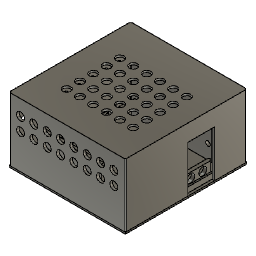
power hotbed caddy v6 (Autodesk Fusion 360 design; units mm, degrees)
Autodesk Fusion 360 part; units mm, degrees
sketch "OUTLINE" plane through (0, 0, 0) normal (0, 0, 1) x (1, 0, 0)
  line L0 (42, -44) -> (-42, -44)
  line L1 (-42, -44) -> (-42, 44)
  line L2 (-42, 44) -> (42, 44)
  line L3 (42, 44) -> (42, -44)
  line L4 (42, -44) -> (-42, 44) construction
  line L5 (-42, -44) -> (42, 44) construction
  line L6 (-42, -44) -> (-40.4, -44) construction
  line L7 (-40.4, -44) -> (-40.4, 44) construction
  line L8 (-40.4, 44) -> (-42, 44) construction
  line L9 (-42, 44) -> (-42, -44) construction
  line L10 (-42, -44) -> (42, -44) construction
  line L11 (42, -44) -> (42, -42.4) construction
  line L12 (42, -42.4) -> (-42, -42.4) construction
  line L13 (-42, -42.4) -> (-42, -44) construction
  line L14 (42, -44) -> (40.4, -44) construction
  line L15 (40.4, -44) -> (40.4, 44) construction
  line L16 (40.4, 44) -> (42, 44) construction
  line L17 (42, 44) -> (42, -44) construction
  line L18 (42, 44) -> (-42, 44) construction
  line L19 (-42, 44) -> (-42, 42.4) construction
  line L20 (-42, 42.4) -> (42, 42.4) construction
  line L21 (42, 42.4) -> (42, 44) construction
  line L22 (40.4, 42.3238) -> (-40.4, 42.3238)
  line L23 (-40.4, 42.3238) -> (-40.4, -42.3238)
  line L24 (-40.4, -42.3238) -> (40.4, -42.3238)
  line L25 (40.4, -42.3238) -> (40.4, 42.3238)
  line L26 (40.4, 42.3238) -> (-40.4, -42.3238) construction
  line L27 (-40.4, 42.3238) -> (40.4, -42.3238) construction
  line L28 (-40.4, -42.3238) -> (40.4, -42.3238) construction
  line L29 (40.4, -42.3238) -> (40.4, -34.3238) construction
  line L30 (40.4, -34.3238) -> (-40.4, -34.3238) construction
  line L31 (-40.4, -34.3238) -> (-40.4, -42.3238) construction
  line L32 (-40.4, 42.3238) -> (40.4, 42.3238) construction
  line L33 (40.4, 42.3238) -> (40.4, 34.3238) construction
  line L34 (40.4, 34.3238) -> (-40.4, 34.3238) construction
  line L35 (-40.4, 34.3238) -> (-40.4, 42.3238) construction
  line L36 (-29.5478, 34.3238) -> (30.4522, 34.3238)
  line L37 (30.4522, 34.3238) -> (30.4522, 32.3238)
  line L38 (30.4522, 32.3238) -> (-29.5478, 32.3238)
  line L39 (-29.5478, 32.3238) -> (-29.5478, 34.3238)
  line L40 (-29.5478, -34.3238) -> (14.4522, -34.3238)
  line L41 (14.4522, -34.3238) -> (14.4522, -32.3238)
  line L42 (14.4522, -32.3238) -> (-29.5478, -32.3238)
  line L43 (-29.5478, -32.3238) -> (-29.5478, -34.3238)
  line L44 (-36.5645, -28.9894) -> (-33.9645, -28.9894)
  line L45 (-33.9645, -28.9894) -> (-33.9645, 26.0106)
  line L46 (-33.9645, 26.0106) -> (-36.5645, 26.0106)
  line L47 (-36.5645, 26.0106) -> (-36.5645, -28.9894)
  line L48 (34.4355, 26.0106) -> (34.4355, -28.9894)
  line L49 (34.4355, -28.9894) -> (37.0355, -28.9894)
  line L50 (37.0355, -28.9894) -> (37.0355, 26.0106)
  line L51 (37.0355, 26.0106) -> (34.4355, 26.0106)
  line L52 (43.6, -45.6) -> (-43.6, -45.6)
  line L53 (-43.6, -45.6) -> (-43.6, 45.6)
  line L54 (-43.6, 45.6) -> (43.6, 45.6)
  line L55 (43.6, 45.6) -> (43.6, -45.6)
  line L56 (43.6, -45.6) -> (-43.6, 45.6) construction
  line L57 (-43.6, -45.6) -> (43.6, 45.6) construction
  dimension "d1" = 84
  dimension "d2" = 88
  dimension "d3" = 1.6
  dimension "d4" = 1.6
  dimension "d5" = 1.6
  dimension "d6" = 1.6
  dimension "d7" = 8
  dimension "d8" = 80.8
  dimension "d9" = 8
  dimension "d10" = 60
  dimension "d11" = 2
  dimension "d12" = 44
  dimension "d13" = 2
  dimension "d14" = 80.8
  dimension "d15" = 2.6
  dimension "d16" = 55
  dimension "d17" = 2.6
  dimension "d18" = 55
  dimension "d47" = 1.6
  dimension "d48" = 1.6
  constraint horizontal L0
  constraint perpendicular L0 L1
  constraint parallel L0 L2
  constraint parallel L1 L3
  constraint coincident L4 origin
  constraint coincident L5 origin
  constraint horizontal L6
  constraint vertical L7
  constraint horizontal L8
  constraint vertical L9
  constraint horizontal L10
  constraint vertical L11
  constraint horizontal L12
  constraint vertical L13
  constraint horizontal L14
  constraint vertical L15
  constraint horizontal L16
  constraint vertical L17
  constraint horizontal L18
  constraint vertical L19
  constraint horizontal L20
  constraint vertical L21
  constraint horizontal L22
  constraint perpendicular L22 L23
  constraint parallel L22 L24
  constraint parallel L23 L25
  constraint coincident L5 L22.start
  constraint coincident L15 L22.start
  constraint coincident L26 origin
  constraint coincident L27 origin
  constraint horizontal L28
  constraint vertical L29
  constraint horizontal L30
  constraint vertical L31
  constraint horizontal L32
  constraint vertical L33
  constraint horizontal L34
  constraint vertical L35
  constraint horizontal L36
  constraint vertical L37
  constraint horizontal L38
  constraint vertical L39
  constraint coincident L34 L36.start
  constraint horizontal L40
  constraint vertical L41
  constraint horizontal L42
  constraint vertical L43
  constraint coincident L30 L40.start
  constraint horizontal L44
  constraint vertical L45
  constraint horizontal L46
  constraint vertical L47
  constraint horizontal L49
  constraint vertical L50
  constraint horizontal L51
  constraint vertical L48
  constraint horizontal L52
  constraint perpendicular L52 L53
  constraint parallel L52 L54
  constraint parallel L53 L55
  constraint coincident L56 origin
  constraint coincident L57 origin
  measures "d1" distance of L1.end L2.end
  measures "d2" distance of L0.end L1.end
  measures "d3" distance of L0.end L6.end
  measures "d4" distance of L0.end L12.end
  measures "d5" distance of L0.start L14.end
  measures "d6" distance of L2.end L20.end
  measures "d7" distance of L23.end L30.end
  measures "d8" distance of L22.end L22.start
  measures "d9" distance of L22.end L34.end
  measures "d10" distance of L36.start L36.end
  measures "d11" distance of L36.start L38.end
  measures "d12" distance of L40.start L40.end
  measures "d13" distance of L40.start L42.end
  measures "d14" distance of L29.end L30.end
  measures "d15" distance of L44.start L44.end
  measures "d16" distance of L44.start L46.end
  measures "d17" distance of L49.end L48.end
  measures "d18" distance of L48.end L48.start
  measures "d47" distance of L3 L55
  measures "d48" distance of L10 L52
extrude "Extrude1" add sketch "OUTLINE" against normal blind 1 contours L0 L1 L2 L3 | L22 L23 L24 L25 | L36 L37 L38 L39 | L40 L41 L42 L43 | L44 L45 L46 L47 | L48 L49 L50 L51 makes body 1
extrude "Extrude2" add sketch "OUTLINE" along normal blind 44 contours L36 L37 L38 L39 bodies 1
extrude "Extrude3" add sketch "OUTLINE" along normal blind 24 contours L40 L41 L42 L43 bodies 1
extrude "Extrude4" add sketch "OUTLINE" along normal blind 8 contours L48 L49 L50 L51 bodies 1
extrude "Extrude5" add sketch "OUTLINE" along normal blind 8 contours L44 L45 L46 L47 bodies 1
hole "Hole1" at (-36.5645, 19.0841, 3.9854) direction (1, 0, 0) diameter 6 depth 100 tip angle 118 bodies 1
hole "Hole2" at (-36.5645, 10.019, 4.0988) direction (1, 0, 0) diameter 6 depth 100 tip angle 118 bodies 1
hole "Hole3" at (-36.5645, 1.1791, 4.164) direction (1, 0, 0) diameter 6 depth 100 tip angle 118 bodies 1
hole "Hole4" at (-36.5645, -7.2432, 4.1822) direction (1, 0, 0) diameter 6 depth 100 tip angle 118 bodies 1
hole "Hole5" at (-36.5645, -14.9986, 4.2656) direction (1, 0, 0) diameter 6 depth 100 tip angle 118 bodies 1
hole "Hole6" at (-36.5645, -22.5039, 4.0988) direction (1, 0, 0) diameter 6 depth 100 tip angle 118 bodies 1
extrude "Extrude6" add sketch "OUTLINE" along normal blind 2 contours L0 L1 L2 L3 bodies 1
extrude "Extrude7" add sketch "OUTLINE" along normal blind 46 separate body contours L52 L53 L54 L55 makes body 2
extrude "Extrude8" add sketch "OUTLINE" against normal blind 1 contours L52 L53 L54 L55 bodies 1
extrude "Extrude9" cut 1 faces at (-42, -14.6667, 0.6667) along direction (1, 0, 0) blind 0.4 on bodies 1 bodies 1
extrude "Extrude10" cut 1 faces at (14.1333, -44, 0.6667) along direction (0, 1, 0) blind 0.4 on bodies 1 bodies 1
extrude "Extrude12" cut 1 faces at (42, 14.8, 0.6667) along direction (-1, 0, 0) blind 0.4 on bodies 1 bodies 1
extrude "Extrude13" cut 1 faces at (-13.8667, 44, 0.6667) along direction (0, -1, 0) blind 0.4 on bodies 1 bodies 1
chamfer "Chamfer1" distance 1 angle 45 1 edges at (41.6, -43.6, 1) on bodies 1
chamfer "Chamfer2" distance 1 angle 45 1 edges at (-41.6, -43.6, 1) on bodies 1
chamfer "Chamfer3" distance 1 angle 45 1 edges at (-41.6, 43.6, 1) on bodies 1
chamfer "Chamfer4" distance 1 angle 45 1 edges at (41.6, 43.6, 1) on bodies 1
chamfer "Chamfer5" distance 1 angle 45 2 edges at (37.0355, 26.0106, 4) (34.4355, 26.0106, 4) on bodies 1
chamfer "Chamfer6" distance 1 angle 45 2 edges at (37.0355, -28.9894, 4) (34.4355, -28.9894, 4) on bodies 1
chamfer "Chamfer7" distance 1 angle 45 4 edges at (-33.9645, -28.9894, 4) (-36.5645, -28.9894, 4) (-36.5645, 26.0106, 4) (-33.9645, 26.0106, 4) on bodies 1
sketch "TOP" plane through (0, 0, 46) normal (0, 0, 1) x (-1, 0, 0)
  line L0 (42, -44) -> (-42, -44)
  line L1 (-42, -44) -> (-42, 44)
  line L2 (-42, 44) -> (42, 44)
  line L3 (42, 44) -> (42, -44)
  line L4 (-43.6, -45.6) -> (43.6, -45.6)
  line L5 (43.6, -45.6) -> (43.6, 45.6)
  line L6 (43.6, 45.6) -> (-43.6, 45.6)
  line L7 (-43.6, 45.6) -> (-43.6, -45.6)
  line L8 (43.6, -45.6) -> (-43.6, -45.6)
  line L9 (-43.6, -45.6) -> (-43.6, 45.6)
  line L10 (-43.6, 45.6) -> (43.6, 45.6)
  line L11 (43.6, 45.6) -> (43.6, -45.6)
  constraint horizontal L8
  constraint vertical L9
  constraint horizontal L10
  constraint vertical L11
  constraint coincident L6.end L7.start
  constraint coincident L4.end L5.start
extrude "Extrude14" add sketch "TOP" along normal blind 1.2 contours L0 L1 L2 L3 | L4 L5 L6 L7 L8 L9 L10 L11 bodies 2
sketch "CABLE HOLES" plane through (-43.6, 0, 0) normal (-1, 0, 0) x (0, -1, 0)
  line L0 (-45.6, 0) -> (45.6, 0)
  line L1 (45.6, 0) -> (45.6, 47.2)
  line L2 (45.6, 47.2) -> (-45.6, 47.2)
  line L3 (-45.6, 47.2) -> (-45.6, 0)
  line L4 (-21.3761, 35, -87.2) -> (-1.3761, 35, -87.2)
  line L5 (-1.3761, 35, -87.2) -> (-1.3761, 0, -87.2)
  line L6 (-1.3761, 0, -87.2) -> (-21.3761, 0, -87.2)
  line L7 (-21.3761, 0, -87.2) -> (-21.3761, 35, -87.2)
  dimension "d74" = 20
  dimension "d75" = 35
extrude "Extrude15" [suppressed]
sketch "BUCK CONVERTER MOUNTING" plane through (0, -34.3238, 0) normal (0, -1, 0) x (1, 0, 0)
  line L0 (-29.5478, 0) -> (14.4522, 0)
  line L1 (14.4522, 0) -> (14.4522, 24)
  line L2 (14.4522, 24) -> (-29.5478, 24)
  line L3 (-29.5478, 24) -> (-29.5478, 0)
  line L4 (-29.5478, 24) -> (-28.5478, 24) construction
  line L5 (-28.5478, 24) -> (-28.5478, 4) construction
  line L6 (-28.5478, 4) -> (-29.5478, 4) construction
  line L7 (-29.5478, 4) -> (-29.5478, 24) construction
  line L8 (14.4522, 24) -> (13.4522, 24) construction
  line L9 (13.4522, 24) -> (13.4522, 4) construction
  line L10 (13.4522, 4) -> (14.4522, 4) construction
  line L11 (14.4522, 4) -> (14.4522, 24) construction
  line L12 (-29.5478, 24) -> (-24.5478, 24) construction
  line L13 (-24.5478, 24) -> (-24.5478, 23) construction
  line L14 (-24.5478, 23) -> (-29.5478, 23) construction
  line L15 (-29.5478, 23) -> (-29.5478, 24) construction
  line L16 (-29.5478, 4) -> (-24.5478, 4) construction
  line L17 (-24.5478, 4) -> (-24.5478, 5) construction
  line L18 (-24.5478, 5) -> (-29.5478, 5) construction
  line L19 (-29.5478, 5) -> (-29.5478, 4) construction
  line L20 (14.4522, 24) -> (9.4522, 24) construction
  line L21 (9.4522, 24) -> (9.4522, 23) construction
  line L22 (9.4522, 23) -> (14.4522, 23) construction
  line L23 (14.4522, 23) -> (14.4522, 24) construction
  line L24 (14.4522, 4) -> (9.4522, 4) construction
  line L25 (9.4522, 4) -> (9.4522, 5) construction
  line L26 (9.4522, 5) -> (14.4522, 5) construction
  line L27 (14.4522, 5) -> (14.4522, 4) construction
  circle A0 centre (-22.7778, 21.23) radius 1.77
  circle A1 centre (7.6822, 21.23) radius 1.77
  circle A2 centre (7.6822, 6.77) radius 1.77
  circle A3 centre (-22.7778, 6.77) radius 1.77
  dimension "d78" = 1
  dimension "d79" = 20
  dimension "d80" = 1
  dimension "d81" = 20
  dimension "d82" = 5
  dimension "d83" = 1
  dimension "d84" = 5
  dimension "d85" = 1
  dimension "d86" = 5
  dimension "d87" = 1
  dimension "d88" = 5
  dimension "d89" = 1
  dimension "d90" = 1.77
  dimension "d91" = 1.77
  dimension "d92" = 1.77
  dimension "d93" = 1.77
  constraint horizontal L4
  constraint vertical L5
  constraint horizontal L6
  constraint vertical L7
  constraint coincident L2.end L3.start
  constraint horizontal L8
  constraint vertical L9
  constraint horizontal L10
  constraint vertical L11
  constraint coincident L1.end L2.start
  constraint horizontal L12
  constraint vertical L13
  constraint horizontal L14
  constraint vertical L15
  constraint horizontal L16
  constraint vertical L17
  constraint horizontal L18
  constraint vertical L19
  constraint horizontal L20
  constraint vertical L21
  constraint horizontal L22
  constraint vertical L23
  constraint horizontal L24
  constraint vertical L25
  constraint horizontal L26
  constraint vertical L27
  constraint tangent L14 A0
  constraint tangent L13 A0
  constraint tangent L21 A1
  constraint tangent L22 A1
  constraint tangent L25 A2
  constraint tangent L26 A2
  constraint tangent L17 A3
  constraint tangent L18 A3
  measures "d78" distance of L2.end L4.end
  measures "d79" distance of L2.end L6.end
  measures "d80" distance of L1.end L8.end
  measures "d81" distance of L1.end L10.end
  measures "d82" distance of L2.end L12.end
  measures "d83" distance of L2.end L14.end
  measures "d84" distance of L6.end L16.end
  measures "d85" distance of L6.end L18.end
  measures "d86" distance of L1.end L20.end
  measures "d87" distance of L1.end L22.end
  measures "d88" distance of L10.end L24.end
  measures "d89" distance of L10.end L26.end
  measures "d90" radius of A0
  measures "d91" radius of A1
  measures "d92" radius of A2
  measures "d93" radius of A3
sketch "HOTBED POWER MODULE MOUNTING" plane through (0, 32.3238, 0) normal (0, -1, 0) x (1, 0, 0)
  line L0 (-29.5478, 0) -> (30.4522, 0)
  line L1 (30.4522, 0) -> (30.4522, 44)
  line L2 (30.4522, 44) -> (-29.5478, 44)
  line L3 (-29.5478, 44) -> (-29.5478, 0)
  line L4 (-29.5478, 44) -> (-28.5478, 44) construction
  line L5 (-28.5478, 44) -> (-28.5478, 4) construction
  line L6 (-28.5478, 4) -> (-29.5478, 4) construction
  line L7 (-29.5478, 4) -> (-29.5478, 44) construction
  line L8 (30.4522, 44) -> (29.4522, 44) construction
  line L9 (29.4522, 44) -> (29.4522, 4) construction
  line L10 (29.4522, 4) -> (30.4522, 4) construction
  line L11 (30.4522, 4) -> (30.4522, 44) construction
  line L12 (-29.5478, 44) -> (-28.5478, 44) construction
  line L13 (-28.5478, 44) -> (-28.5478, 39) construction
  line L14 (-28.5478, 39) -> (-29.5478, 39) construction
  line L15 (-29.5478, 39) -> (-29.5478, 44) construction
  line L16 (30.4522, 44) -> (29.4522, 44) construction
  line L17 (29.4522, 44) -> (29.4522, 39) construction
  line L18 (29.4522, 39) -> (30.4522, 39) construction
  line L19 (30.4522, 39) -> (30.4522, 44) construction
  line L20 (30.4522, 4) -> (29.4522, 4) construction
  line L21 (29.4522, 4) -> (29.4522, 9) construction
  line L22 (29.4522, 9) -> (30.4522, 9) construction
  line L23 (30.4522, 9) -> (30.4522, 4) construction
  line L24 (-29.5478, 4) -> (-28.5478, 4) construction
  line L25 (-28.5478, 4) -> (-28.5478, 9) construction
  line L26 (-28.5478, 9) -> (-29.5478, 9) construction
  line L27 (-29.5478, 9) -> (-29.5478, 4) construction
  line L28 (-28.5478, 24) -> (-28.5478, 4)
  circle A0 centre (-26.7778, 10.77) radius 1.77
  circle A1 centre (27.6822, 10.77) radius 1.77
  circle A2 centre (-26.7778, 37.23) radius 1.77
  circle A3 centre (27.6822, 37.23) radius 1.77
  dimension "d94" = 1
  dimension "d95" = 40
  dimension "d96" = 1
  dimension "d97" = 40
  dimension "d98" = 1
  dimension "d99" = 5
  dimension "d100" = 1
  dimension "d101" = 5
  dimension "d102" = 1
  dimension "d103" = 5
  dimension "d104" = 1
  dimension "d105" = 5
  dimension "d106" = 1.77
  dimension "d107" = 1.77
  dimension "d108" = 1.77
  dimension "d109" = 1.77
  constraint horizontal L4
  constraint vertical L5
  constraint horizontal L6
  constraint vertical L7
  constraint coincident L2.end L3.start
  constraint horizontal L8
  constraint vertical L9
  constraint horizontal L10
  constraint vertical L11
  constraint coincident L1.end L2.start
  constraint horizontal L12
  constraint vertical L13
  constraint horizontal L14
  constraint vertical L15
  constraint horizontal L16
  constraint vertical L17
  constraint horizontal L18
  constraint vertical L19
  constraint horizontal L20
  constraint vertical L21
  constraint horizontal L22
  constraint vertical L23
  constraint horizontal L24
  constraint vertical L25
  constraint horizontal L26
  constraint vertical L27
  constraint tangent L28 A0
  constraint tangent L26 A0
  constraint tangent L21 A1
  constraint tangent L22 A1
  constraint tangent L14 A2
  constraint tangent L5 A2
  constraint tangent L9 A3
  constraint tangent L18 A3
  measures "d94" distance of L2.end L4.end
  measures "d95" distance of L2.end L6.end
  measures "d96" distance of L1.end L8.end
  measures "d97" distance of L1.end L10.end
  measures "d98" distance of L2.end L4.end
  measures "d99" distance of L2.end L14.end
  measures "d100" distance of L1.end L8.end
  measures "d101" distance of L1.end L18.end
  measures "d102" distance of L10.end L9.end
  measures "d103" distance of L10.end L22.end
  measures "d104" distance of L6.end L5.end
  measures "d105" distance of L6.end L26.end
  measures "d106" radius of A0
  measures "d107" radius of A1
  measures "d108" radius of A2
  measures "d109" radius of A3
extrude "Extrude16" cut sketch "HOTBED POWER MODULE MOUNTING" against normal blind 6 contours A0 | A1 | A2 | A3 bodies 1
extrude "Extrude17" cut sketch "BUCK CONVERTER MOUNTING" against normal blind 9 contours A0 | A1 | A2 | A3 bodies 1
sketch "SIDE HOLES (1)" plane through (-43.6, 0, 0) normal (-1, 0, 0) x (0, -1, 0)
  line L0 (-45.6, 0) -> (45.6, 0)
  line L1 (45.6, 0) -> (45.6, 47.2)
  line L2 (45.6, 47.2) -> (-45.6, 47.2)
  line L3 (-45.6, 47.2) -> (-45.6, 0)
  circle A0 centre (-34, 36) radius 3
  circle A1 centre (-34, 26) radius 3
  circle A2 centre (-24, 26) radius 3
  circle A3 centre (-24, 36) radius 3
  circle A4 centre (-14, 26) radius 3
  circle A5 centre (-14, 36) radius 3
  circle A6 centre (-4, 36) radius 3
  circle A7 centre (-4, 26) radius 3
  circle A8 centre (6, 36) radius 3
  circle A9 centre (6, 26) radius 3
  circle A10 centre (16, 26) radius 3
  circle A11 centre (16, 36) radius 3
  circle A12 centre (26, 36) radius 3
  circle A13 centre (26, 26) radius 3
  circle A14 centre (36, 26) radius 3
  circle A15 centre (36, 36) radius 3
  dimension "d114" = 6
  dimension "d115" = 6
  dimension "d116" = 6
  dimension "d117" = 6
  dimension "d118" = 6
  dimension "d119" = 6
  dimension "d120" = 6
  dimension "d121" = 6
  dimension "d122" = 6
  dimension "d123" = 6
  dimension "d124" = 6
  dimension "d125" = 6
  dimension "d126" = 6
  dimension "d127" = 6
  dimension "d128" = 6
  dimension "d129" = 6
  measures "d114" diameter of A0
  measures "d115" diameter of A1
  measures "d116" diameter of A3
  measures "d117" diameter of A2
  measures "d118" diameter of A5
  measures "d119" diameter of A4
  measures "d120" diameter of A6
  measures "d121" diameter of A7
  measures "d122" diameter of A8
  measures "d123" diameter of A9
  measures "d124" diameter of A11
  measures "d125" diameter of A10
  measures "d126" diameter of A12
  measures "d127" diameter of A13
  measures "d128" diameter of A15
  measures "d129" diameter of A14
extrude "Extrude18" cut sketch "SIDE HOLES (1)" against normal blind 7 contours A0 | A1 | A2 | A3 | A4 | A5 | A6 | A7 | A8 | A9 | A10 | A11 | A12 | A13 | A14 | A15 bodies 2
sketch "OTHER SIDE HOLES" plane through (0, -45.6, 0) normal (0, -1, 0) x (1, 0, 0)
  line L0 (-43.6, 0) -> (43.6, 0)
  line L1 (43.6, 0) -> (43.6, 47.2)
  line L2 (43.6, 47.2) -> (-43.6, 47.2)
  line L3 (-43.6, 47.2) -> (-43.6, 0)
  circle A0 centre (-35, 36) radius 3
  circle A1 centre (-25, 36) radius 3
  circle A2 centre (-15, 36) radius 3
  circle A3 centre (-5, 36) radius 3
  circle A4 centre (5, 36) radius 3
  circle A5 centre (15, 36) radius 3
  circle A6 centre (25, 36) radius 3
  circle A7 centre (35, 36) radius 3
  circle A8 centre (-35, 26) radius 3
  circle A9 centre (-25, 26) radius 3
  circle A10 centre (-15, 26) radius 3
  circle A11 centre (-5, 26) radius 3
  circle A12 centre (5, 26) radius 3
  circle A13 centre (15, 26) radius 3
  circle A14 centre (25, 26) radius 3
  circle A15 centre (35, 26) radius 3
  dimension "d132" = 6
  dimension "d133" = 6
  dimension "d134" = 6
  dimension "d135" = 6
  dimension "d136" = 6
  dimension "d137" = 6
  dimension "d138" = 6
  dimension "d139" = 6
  dimension "d140" = 6
  dimension "d141" = 6
  dimension "d142" = 6
  dimension "d143" = 6
  dimension "d144" = 6
  dimension "d145" = 6
  dimension "d146" = 6
  dimension "d147" = 6
  measures "d132" diameter of A0
  measures "d133" diameter of A1
  measures "d134" diameter of A2
  measures "d135" diameter of A3
  measures "d136" diameter of A4
  measures "d137" diameter of A5
  measures "d138" diameter of A6
  measures "d139" diameter of A7
  measures "d140" diameter of A8
  measures "d141" diameter of A9
  measures "d142" diameter of A10
  measures "d143" diameter of A11
  measures "d144" diameter of A12
  measures "d145" diameter of A13
  measures "d146" diameter of A14
  measures "d147" diameter of A15
extrude "Extrude19" cut sketch "OTHER SIDE HOLES" against normal blind 118 contours A0 | A1 | A2 | A3 | A4 | A5 | A6 | A7 | A8 | A9 | A10 | A11 | A12 | A13 | A14 | A15 bodies 2
chamfer "Chamfer8" distance 1 angle 45 2 edges at (43.6, -45.6, 23.6) (43.6, 45.6, 23.6) on bodies 2
sketch "top holes" plane through (0, 0, 47.2) normal (0, 0, 1) x (-1, 0, 0)
  line L0 (-42.6, -45.6) -> (43.6, -45.6)
  line L1 (43.6, -45.6) -> (43.6, 45.6)
  line L2 (43.6, 45.6) -> (-42.6, 45.6)
  line L3 (-43.6, 44.6) -> (-43.6, -44.6)
  circle A0 centre (-26, -18) radius 3
  circle A1 centre (-26, -8) radius 3
  circle A2 centre (-26, 2) radius 3
  circle A3 centre (-26, 12) radius 3
  circle A4 centre (-26, 22) radius 3
  circle A5 centre (-16, -8) radius 3
  circle A6 centre (-16, -18) radius 3
  circle A7 centre (-16, 2) radius 3
  circle A8 centre (-16, 12) radius 3
  circle A9 centre (-16, 22) radius 3
  circle A10 centre (4, -18) radius 3
  circle A11 centre (4, -8) radius 3
  circle A12 centre (4, 2) radius 3
  circle A13 centre (4, 12) radius 3
  circle A14 centre (4, 22) radius 3
  circle A15 centre (-6, 22) radius 3
  circle A16 centre (-6, 12) radius 3
  circle A17 centre (-6, 2) radius 3
  circle A18 centre (-6, -8) radius 3
  circle A19 centre (-6, -18) radius 3
  circle A20 centre (14, -18) radius 3
  circle A21 centre (14, -8) radius 3
  circle A22 centre (14, 2) radius 3
  circle A23 centre (14, 12) radius 3
  circle A24 centre (14, 22) radius 3
  circle A25 centre (24, 22) radius 3
  circle A26 centre (24, 12) radius 3
  circle A27 centre (24, 2) radius 3
  circle A28 centre (24, -8) radius 3
  circle A29 centre (24, -18) radius 3
  line L4 (-43.6, -44.6) -> (-42.6, -45.6)
  line L5 (-42.6, 45.6) -> (-43.6, 44.6)
  dimension "d151" = 6
  dimension "d152" = 6
  dimension "d153" = 6
  dimension "d154" = 6
  dimension "d155" = 6
  dimension "d156" = 6
  dimension "d157" = 6
  dimension "d158" = 6
  dimension "d159" = 6
  dimension "d160" = 6
  dimension "d161" = 10
  dimension "d162" = 10
  dimension "d163" = 10
  dimension "d164" = 10
  dimension "d165" = 10
  dimension "d166" = 6
  dimension "d167" = 6
  dimension "d168" = 6
  dimension "d169" = 6
  dimension "d170" = 6
  dimension "d171" = 6
  dimension "d172" = 6
  dimension "d173" = 6
  dimension "d174" = 6
  dimension "d175" = 6
  dimension "d176" = 10
  dimension "d177" = 10
  dimension "d178" = 10
  dimension "d179" = 10
  dimension "d180" = 10
  dimension "d181" = 6
  dimension "d182" = 6
  dimension "d183" = 6
  dimension "d184" = 6
  dimension "d185" = 6
  dimension "d186" = 6
  dimension "d187" = 6
  dimension "d188" = 6
  dimension "d189" = 6
  dimension "d190" = 6
  dimension "d191" = 10
  dimension "d192" = 10
  dimension "d193" = 10
  dimension "d194" = 10
  dimension "d195" = 10
  measures "d151" diameter of A0
  measures "d152" diameter of A1
  measures "d153" diameter of A2
  measures "d154" diameter of A3
  measures "d155" diameter of A4
  measures "d156" diameter of A6
  measures "d157" diameter of A5
  measures "d158" diameter of A7
  measures "d159" diameter of A8
  measures "d160" diameter of A9
  measures "d161" distance of A0.centre A6.centre
  measures "d162" distance of A1.centre A5.centre
  measures "d163" distance of A2.centre A7.centre
  measures "d164" distance of A3.centre A8.centre
  measures "d165" distance of A4.centre A9.centre
  measures "d166" diameter of A19
  measures "d167" diameter of A18
  measures "d168" diameter of A17
  measures "d169" diameter of A16
  measures "d170" diameter of A15
  measures "d171" diameter of A10
  measures "d172" diameter of A11
  measures "d173" diameter of A12
  measures "d174" diameter of A13
  measures "d175" diameter of A14
  measures "d176" distance of A19.centre A10.centre
  measures "d177" distance of A18.centre A11.centre
  measures "d178" distance of A12.centre A17.centre
  measures "d179" distance of A16.centre A13.centre
  measures "d180" distance of A15.centre A14.centre
  measures "d181" diameter of A20
  measures "d182" diameter of A21
  measures "d183" diameter of A22
  measures "d184" diameter of A23
  measures "d185" diameter of A24
  measures "d186" diameter of A29
  measures "d187" diameter of A28
  measures "d188" diameter of A27
  measures "d189" diameter of A26
  measures "d190" diameter of A25
  measures "d191" distance of A20.centre A29.centre
  measures "d192" distance of A21.centre A28.centre
  measures "d193" distance of A27.centre A22.centre
  measures "d194" distance of A23.centre A26.centre
  measures "d195" distance of A24.centre A25.centre
extrude "Extrude20" cut sketch "top holes" against normal blind 2 contours A0 | A1 | A2 | A3 | A4 | A5 | A6 | A7 | A8 | A9 | A10 | A11 | A12 | A13 | A14 | A15 | A16 | A17 | A18 | A19 | A20 | A21 | A22 | A23 | A24 | A25 | A26 | A27 | A28 | A29 bodies 2
extrude "Extrude21" cut sketch "CABLE HOLES" along normal blind 2 contours L4 L5 L6 L7 in plane through (43.6, 0, 0) normal (-1, 0, 0) bodies 2
sketch "Sketch10" plane through (-43.6, 0, 0) normal (-1, 0, 0) x (0, -1, 0)
  circle A0 centre (-14, 36) radius 3
  circle A1 centre (-14, 26) radius 3
  circle A2 centre (26, 26) radius 3
  circle A3 centre (16, 36) radius 3
  circle A4 centre (26, 36) radius 3
  circle A5 centre (16, 26) radius 3
  circle A6 centre (-24, 26) radius 3
  circle A7 centre (-4, 36) radius 3
  circle A8 centre (-24, 36) radius 3
  circle A9 centre (-4, 26) radius 3
  circle A10 centre (36, 26) radius 3
  circle A11 centre (-34, 36) radius 3
  circle A12 centre (36, 36) radius 3
  circle A13 centre (6, 26) radius 3
  circle A14 centre (-34, 26) radius 3
  circle A15 centre (6, 36) radius 3
  line L0 (-45.6, 0) -> (45.6, 0)
  line L1 (45.6, 0) -> (45.6, 47.2)
  line L2 (45.6, 47.2) -> (-45.6, 47.2)
  line L3 (-45.6, 47.2) -> (-45.6, 0)
  line L4 (-8, 0) -> (2, 0)
  line L5 (2, 0) -> (2, 15)
  line L6 (2, 15) -> (-8, 15)
  line L7 (-8, 15) -> (-8, 0)
  dimension "d200" = 10
  dimension "d201" = 15
  constraint horizontal L4
  constraint vertical L5
  constraint horizontal L6
  constraint vertical L7
  constraint coincident L0 L4.start
  measures "d200" distance of L4.start L4.end
  measures "d201" distance of L4.start L6.end
extrude "Extrude22" cut sketch "Sketch10" against normal blind 6 contours L0 L4 L5 L6 L7 bodies 2
extrude "Extrude23" [suppressed]
extrude "Extrude24" [suppressed]
extrude "Extrude25" [suppressed]
extrude "Extrude26" [suppressed]
extrude "Extrude27" [suppressed]
extrude "Extrude28" add 1 faces at (-14.5333, -15.2, -1) along direction (0, 0, -1) blind 0.2 on bodies 1 bodies 1
extrude "Extrude29" add 1 faces at (-12.0929, -34.3238, 11.846) along direction (0, -1, 0) blind 0.2 on bodies 1 bodies 1
extrude "Extrude30" add 1 faces at (-8.0929, 34.3238, 28.154) along direction (0, 1, 0) blind 0.2 on bodies 1 bodies 1
extrude "Extrude31" add 1 faces at (13.4667, -43.1746, 2) along direction (0, 0, 1) blind 2 on bodies 1 bodies 1
extrude "Extrude32" add 1 faces at (1.5919, 44, 7.6695) along direction (0, -1, 0) blind 0.3 on bodies 2 bodies 2
extrude "Extrude33" add 1 faces at (42, -28.8746, 27) along direction (-1, 0, 0) blind 0.3 on bodies 2 bodies 2
extrude "Extrude34" add 1 faces at (-1.6919, -44, 7.6695) along direction (0, 1, 0) blind 0.3 on bodies 2 bodies 2
extrude "Extrude35" add 1 faces at (-42, -23.8253, 7.6695) along direction (1, 0, 0) blind 0.3 on bodies 2 bodies 2
extrude "Extrude36" add 1 faces at (-1.5919, 37.3972, 47.2) along direction (0, 0, 1) blind 0.3 on bodies 2 bodies 2
chamfer "Chamfer9" distance 1 angle 45 1 edges at (-43.6, -45.6, 23.75) on bodies 2
chamfer "Chamfer10" distance 1 angle 45 1 edges at (-43.6, 45.6, 23.75) on bodies 2
named bodies: "BOTTOM PLATE", "CASE (1)"
